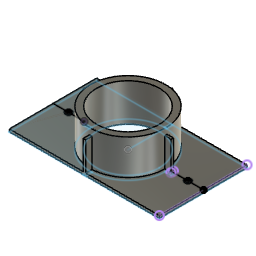
sosten de caños v4 (Autodesk Fusion 360 design; units mm, degrees)
Autodesk Fusion 360 part; units mm, degrees
note: some values were not read from the file. Set by a fixed rule: which sketch regions a step uses.
sketch "Boceto1" plane through (0, 0, 0) normal (0, 0, 1) x (1, 0, 0)
  circle A0 centre (53.322, 1.6797) radius 25
  circle A1 centre (53.322, 1.6797) radius 30
  line L0 (53.322, 36.6797) -> (113.322, 36.6797)
  line L1 (74.1438, -33.3203) -> (-6.3562, -33.3203)
  line L2 (-6.3562, -33.3203) -> (-6.678, 36.6797)
  line L3 (53.322, 36.6797) -> (-6.678, 36.6797)
  line L4 (53.322, 1.6797) -> (53.322, 36.6797)
  line L5 (113.322, 36.6797) -> (113.322, -33.3203)
  line L6 (113.322, -33.3203) -> (74.1438, -33.3203)
  line L7 (53.322, 31.6797) -> (54.322, 31.6797)
  line L8 (54.322, 31.6797) -> (54.322, 36.6797)
  line L9 (53.322, 31.6797) -> (52.322, 31.6797)
  line L10 (52.322, 31.6797) -> (52.322, 36.6797)
  line L11 (53.6438, -28.3186) -> (54.6438, -28.3186)
  line L12 (54.6438, -28.3186) -> (54.6438, -33.3203)
  line L13 (54.6438, -33.3203) -> (52.6438, -33.3203)
  line L14 (52.6438, -28.3127) -> (52.6438, -33.3203)
  line L15 (83.3203, 1.9993) -> (83.3203, 2.9993)
  line L16 (83.3203, 2.9993) -> (88.3203, 2.9993)
  line L17 (88.3203, 2.9993) -> (88.3203, 0.9993)
  line L18 (88.3203, 0.9993) -> (83.3143, 0.9993)
  line L19 (23.322, 1.6797) -> (18.322, 1.6797)
  line L20 (18.322, 1.6797) -> (18.322, 2.6797)
  line L21 (18.322, 2.6797) -> (23.3386, 2.6797)
  line L22 (18.322, 1.6797) -> (18.322, 0.6797)
  line L23 (18.322, 0.6797) -> (23.3386, 0.6797)
  dimension "d1" = 50
  dimension "d2" = 60
  dimension "d4" = 60
  dimension "d5" = 60
  dimension "d6" = 80.5
  dimension "d7" = 70
  dimension "d16" = 35
  dimension "d28" = 1
  dimension "d29" = 1
  dimension "d32" = 1
  dimension "d33" = 2
  dimension "d34" = 1
  dimension "d35" = 5
  dimension "d36" = 2
  dimension "d37" = 5
  dimension "d38" = 1
  dimension "d39" = 1
  constraint concentric A0 A1
  constraint horizontal L0
  constraint coincident A0.centre A1.centre
  constraint perpendicular L0 L4
  constraint coincident L0.start L3.start
  constraint perpendicular L1 L5
  constraint perpendicular L5 L6
  constraint coincident A1 L7.start
  constraint coincident L4 L7.start
  constraint perpendicular L4 L7
  constraint coincident L0 L8.end
  constraint perpendicular L0 L8
  constraint tangent A1 L9
  constraint coincident L3 L10.end
  constraint perpendicular L3 L10
  constraint coincident A1 L11.start
  constraint parallel L1 L11
  constraint coincident L6 L12.end
  constraint perpendicular L6 L12
  constraint coincident L1 L13.end
  constraint coincident A1 L14.start
  constraint perpendicular L13 L14
  constraint coincident A1 L15.start
  constraint perpendicular L11 L15
  constraint perpendicular L15 L16
  constraint perpendicular L16 L17
  constraint coincident A1 L18.end
  constraint perpendicular L15 L18
  constraint coincident A1 L19.start
  constraint perpendicular L4 L19
  constraint perpendicular L19 L20
  constraint coincident A1 L21.end
  constraint perpendicular L20 L21
  constraint perpendicular L19 L22
  constraint coincident A1 L23.end
  constraint perpendicular L20 L23
  measures "d1" diameter of A0
  measures "d2" diameter of A1
  measures "d4" distance of L0.end L0.start
  measures "d5" distance of L2.end L0.start
  measures "d6" distance of L1.end L1.start
  measures "d7" vertical distance of L1.end L2.end
  measures "d16" distance of A0.centre L0.start
  measures "d28" distance of L7.start L7.end
  measures "d29" distance of L7.start L9.end
  measures "d32" distance of L11.start L11.end
  measures "d33" distance of L12.end L13.end
  measures "d34" distance of L15.start L15.end
  measures "d35" distance of L15.end L16.end
  measures "d36" distance of L16.end L17.end
  measures "d37" distance of L19.start L19.end
  measures "d38" distance of L19.end L20.end
  measures "d39" distance of L19.end L22.end
extrude "Extruir1" add sketch "Boceto1" along normal blind 30 contours A1 makes body 1
sketch "Boceto4" plane through (0, 0, 0) normal (0, 0, 1) x (1, 0, 0)
extrude "Extruir7" add sketch "Boceto1" along normal blind 25 separate body contours L3 L4 L9 L10 | L0 L4 L7 L8 makes body 2
extrude "Extruir8" add sketch "Boceto1" along normal blind 25 contours A1 L15 L16 L17 L18 | A1 L1 L11 L12 L13 L14 | A1 L19 L20 L21 | A1 L19 L22 L23 bodies 1
extrude "Extruir9" add sketch "Boceto1" along normal blind 2 contours A1 L0 L1 L5 L6 L7 L8 L11 L12 L15 L16 L17 L18 | A1 L1 L2 L3 L9 L10 L14 L20 L21 L22 L23 bodies 1 2
sketch "Boceto6" plane through (0, 0, 2) normal (0, 0, 1) x (-1, 0, 0)
  line L0 (-18.322, -0.6797) -> (-18.322, -2.6797)
  line L1 (-18.322, -2.6797) -> (-23.3386, -2.6797)
  arc A0 (-53.322, -31.6797) -> (-23.3386, -2.6797) centre (-53.322, -1.6797) ccw
  line L2 (-53.322, -31.6797) -> (-52.322, -31.6797)
  line L3 (-52.322, -31.6797) -> (-52.322, -36.6797)
  line L4 (-52.322, -36.6797) -> (6.678, -36.6797)
  line L5 (6.678, -36.6797) -> (6.3562, 33.3203)
  line L6 (6.3562, 33.3203) -> (-52.6438, 33.3203)
  line L7 (-52.6438, 33.3203) -> (-52.6438, 28.3127)
  arc A1 (-23.3386, -0.6797) -> (-52.6438, 28.3127) centre (-53.322, -1.6797) ccw
  line L8 (-23.3386, -0.6797) -> (-18.322, -0.6797)
  line L9 (-18.322, -1.6797) -> (6.5171, -1.6797)
  circle A2 centre (-5.9024, -1.6797) radius 2.5
  line L10 (-88.3203, -2.9993) -> (-88.3203, -0.9993)
  line L11 (-113.322, 33.3203) -> (-113.322, -36.6797)
  line L12 (-88.3203, -1.9993) -> (-113.322, -1.9993)
  circle A3 centre (-100.8211, -1.9993) radius 2.5
  point P0 (-18.322, -1.6797)
  dimension "d44" = 5
  dimension "d45" = 5
  constraint coincident P0 L9.start
  constraint midpoint L5 L9.end
  constraint midpoint L9 A2.centre
  constraint midpoint L10 L12.start
  constraint coincident L11 L12.end
  constraint perpendicular L11 L12
  constraint midpoint L12 A3.centre
  measures "d44" diameter of A2
  measures "d45" diameter of A3
hole "Agujero2" at (100.8211, 1.9993, 2) direction (0, 0, -1) diameter 3 depth 10 tip angle 180 bodies 1
hole "Agujero3" at (5.9024, 1.6797, 2) direction (0, 0, -1) diameter 3 depth 10 tip angle 180 bodies 1
equation "d6 = 60 mm + 20.5 mm"
